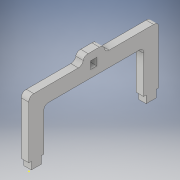
# Autodesk Inventor part: hangar
Saved by Autodesk Inventor 2017.2 (Build 212233000, 233)
## iProperties
Created: 2017-06-16
Part Number: hangar
Material: Generic
Document SubType Name: Modeling
Designer: SandeepSH
Density: 1 g/cm^3
Appearance: Default
Author: SandeepSH
Autodesk Inventor part; units mm, degrees
ref_plane "YZ Plane" through (0, 0, 0) normal (1, 0, 0) x (0, 1, 0)
ref_plane "XZ Plane" through (0, 0, 0) normal (0, 1, 0) x (-1, 0, 0)
ref_plane "XY Plane" through (0, 0, 0) normal (0, 0, 1) x (1, 0, 0)
sketch "Sketch1" plane through (0, 0, 0) normal (1, 0, 0) x (0, 1, 0)
  line L0 (0, 0) -> (29, 0)
  line L1 (29, 0) -> (29, -52)
  line L2 (29, -52) -> (0, -52)
  line L3 (0, -52) -> (0, 0)
  line L4 (0, 0) -> (3, 0)
  line L5 (3, 0) -> (3, -1)
  line L6 (3, -1) -> (0, -1)
  line L7 (0, -1) -> (0, 0)
  line L8 (0, -52) -> (3, -52)
  line L9 (3, -52) -> (3, -51)
  line L10 (3, -51) -> (0, -51)
  line L11 (0, -51) -> (0, -52)
  line L12 (0, -5) -> (20, -5)
  line L13 (20, -5) -> (20, -47)
  line L14 (20, -47) -> (0, -47)
  line L15 (0, -47) -> (0, -5)
  line L16 (29, 0) -> (23, 0)
  line L17 (23, 0) -> (23, -52)
  line L18 (23, -52) -> (29, -52)
  line L19 (29, -52) -> (29, 0)
  line L20 (26, -24.75) -> (26, -27.25)
  line L21 (26, -27.25) -> (23, -27.25)
  line L22 (23, -27.25) -> (23, -24.75)
  line L23 (23, -24.75) -> (26, -24.75)
  line L24 (26, -24.75) -> (23, -27.25) construction
  line L25 (26, -27.25) -> (23, -24.75) construction
  line L26 (3, -5) -> (20, -5)
  line L27 (20, -5) -> (20, -6)
  line L28 (20, -6) -> (3, -6)
  line L29 (3, -6) -> (3, -5)
  line L30 (3, -47) -> (20, -47)
  line L31 (20, -47) -> (20, -46)
  line L32 (20, -46) -> (3, -46)
  line L33 (3, -46) -> (3, -47)
  line L34 (29, 0) -> (26, 0)
  line L35 (26, 0) -> (26, -21.75)
  line L36 (26, -21.75) -> (29, -21.75)
  line L37 (29, -21.75) -> (29, 0)
  line L38 (29, -52) -> (26, -52)
  line L39 (26, -52) -> (26, -30.25)
  line L40 (26, -30.25) -> (29, -30.25)
  line L41 (29, -30.25) -> (29, -52)
  point P0 (24.5, -26)
  dimension "d0" = 29
  dimension "d1" = 52
  dimension "d2" = 3
  dimension "d3" = 1
  dimension "d4" = 3
  dimension "d5" = 1
  dimension "d6" = 20
  dimension "d7" = 4
  dimension "d8" = 4
  dimension "d9" = 6
  dimension "d10" = 2.5
  dimension "d11" = 3
  dimension "d12" = 1
  dimension "d13" = 1
  dimension "d14" = 3
  dimension "d15" = 3
  constraints: 84 end point, 21 parallel, 10 perpendicular, 9 horizontal, 7 point on line, 2 midpoint, 1 collinear
  measures "d0" distance of L1.end L2.end
  measures "d1" distance of L0.end L1.end
  measures "d2" distance of L5.end L6.end
  measures "d3" distance of L4.end L5.end
  measures "d4" distance of L10.end L9.end
  measures "d5" distance of L9.end L8.end
  measures "d6" distance of L13.end L14.end
  measures "d7" distance between parallel lines of L12 L6
  measures "d8" distance between parallel lines of L10 L14
  measures "d9" distance of L18.end L17.end
  measures "d10" distance of L20.start L20.end
  measures "d11" distance of L20.end L21.end
  measures "d12" distance of L26.end L27.end
  measures "d13" distance of L31.end L30.end
  measures "d14" distance between parallel lines of L23 L36
  measures "d15" distance between parallel lines of L40 L21
sketch "Sketch2" plane through (0, 0, 0) normal (1, 0, 0) x (0, 1, 0)
  line L0 (0, 0) -> (29, 0)
  line L1 (29, 0) -> (29, -52)
  line L2 (29, -52) -> (0, -52)
  line L3 (0, -52) -> (0, 0)
  dimension "d16" = 29
  dimension "d17" = 52
  constraints: 8 end point, 2 parallel, 1 horizontal, 1 perpendicular
  measures "d16" distance of L1.end L2.end
  measures "d17" distance of L0.end L1.end
extrude "Extrusion1" add sketch "Sketch2" along normal blind 3
sketch "Sketch3" plane through (3, 0, 0) normal (1, 0, 0) x (0, 0, -1)
  point P0 (0, 0)
extrude "Extrusion2" cut sketch "Sketch1" along normal through all contours L0 L5 L6 L3 | L12 L29 L28 L13 L32 L33 L14 L3 | L0 L1 L36 L35 | L23 L20 L21 L17 | L10 L9 L2 L3 | L1 L2 L39 L40
fillet "Fillet1" radius 2 6 edges at (1.5, 29, -21.75) (1.5, 29, -30.25) (1.5, 26, 0) (1.5, 26, -52) (1.5, 20, -6) (1.5, 20, -46) curvature continuous yes
fillet "Fillet2" radius 2 2 edges at (1.5, 26, -30.25) (1.5, 26, -21.75)
equation "\"d15\" = d14"
body "Solid1"
